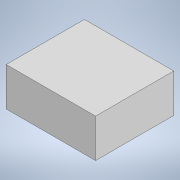
# Autodesk Inventor part: Air Compressor
Saved by Autodesk Inventor 2020 (Build 240168000, 168)
## iProperties
Created: 2021-01-31
Part Number: Air Compressor
Material: Generic
Document SubType Name: Modeling
Designer: magda
Density: 1 g/cm^3
Appearance: Default
Author: magda
Autodesk Inventor part; units mm, degrees
ref_plane "YZ Plane" through (0, 0, 0) normal (1, 0, 0) x (0, 1, 0)
ref_plane "XZ Plane" through (0, 0, 0) normal (0, 1, 0) x (-1, 0, 0)
ref_plane "XY Plane" through (0, 0, 0) normal (0, 0, 1) x (1, 0, 0)
sketch "Sketch1" plane through (0, 0, 0) normal (0, 0, 1) x (1, 0, 0)
  line L0 (-25.4681, 40.284) -> (98.8141, 40.284)
  line L1 (98.8141, 40.284) -> (98.8141, -13.31)
  line L2 (98.8141, -13.31) -> (-25.4681, -13.31)
  line L3 (-25.4681, -13.31) -> (-25.4681, 40.284)
  point P0 (0, 0)
  dimension "d0" = 124.2822
  dimension "d1" = 53.594
  constraints: 8 end point, 2 parallel, 1 horizontal, 1 perpendicular
  measures "d0" distance of L1.end L2.end
  measures "d1" distance of L0.end L1.end
extrude "Extrusion1" add sketch "Sketch1" along normal blind 108.7374
body "Solid1"
